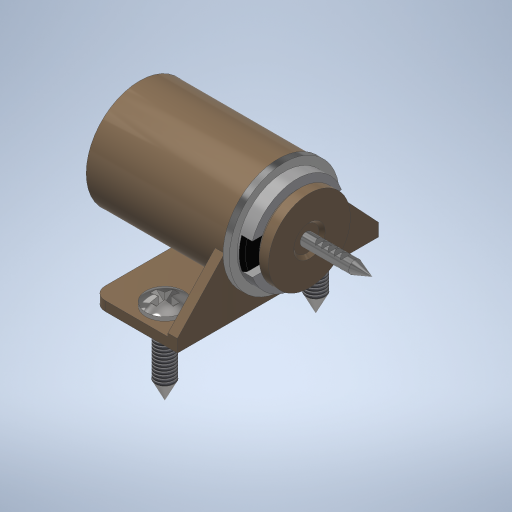
# Autodesk Inventor part: Door fixing magnet
Saved by Autodesk Inventor 2024 (Build 280153000, 153)
## iProperties
Category: Magnets and locks
Created: 2013-04-05
Part Number: Door fixing magnet
Material: Generic
Document SubType Name: Modeling
Designer: G. K.
Authority: Design by UAB Čeli APS
Density: 1 g/cm^3
Description: Door  fixing magnet
Appearance: Default
Mase: 0.0
Author: G. K.
Title: Door fixing magnet
Subject: Magnets
Keywords: door, magnets
Comments: magnet for doors fixing
Revision Number: 1
Autodesk Inventor part; units mm, degrees
sketch "Sketch2" plane through (0, 0, 0) normal (0, 1, 0) x (-1, 0, 0)
  line L0 (0, 0) -> (-25, 0)
  line L1 (0, -7.5) -> (-8, -7.5)
  line L2 (-22, -8.5) -> (0, -8.5)
  line L3 (0, -8.5) -> (0, -7.5)
  line L4 (-8, -7.5) -> (-8, -4)
  line L5 (-8, -4) -> (-2, -4)
  line L6 (-2, -4) -> (-2, 0)
  line L7 (-22, -8.5) -> (-22, -8.75)
  line L8 (-22, -8.75) -> (-23, -8.75)
  line L9 (-23, -8.75) -> (-23, -7.5)
  line L10 (-23, -7.5) -> (-25, -7.5)
  line L11 (-25, -7.5) -> (-25, 0)
  dimension "d0" = 15
  dimension "d2" = 17
  dimension "d3" = 8
  dimension "d4" = 0
  dimension "d5" = 8
  dimension "d6" = 22
  dimension "d7" = 1
  dimension "d8" = 2
  dimension "d9" = 17.5
  dimension "d10" = 15
  dimension "d12" = 23
  constraints: 25 end point, 5 parallel, 5 perpendicular, 1 horizontal, 1 point on line
  measures "d0" diameter of L1 L0
  measures "d2" diameter of L2 L0
  measures "d3" distance between parallel lines of L4 L3
  measures "d4" distance from line of L0.start L3
  measures "d5" diameter of L5 L0
  measures "d6" distance between parallel lines of L7 L3
  measures "d7" distance of L7.end L8.end
  measures "d8" distance of L9.end L10.end
  measures "d9" diameter of L8 L0
  measures "d10" diameter of L10 L0
  measures "d12" distance between parallel lines of L6 L11
revolve "Revolution1" add sketch "Sketch2" angle 360 about axis through (0, 0, 0) along (1, 0, 0)
sketch "Sketch3" plane through (22, 0, 0) normal (-1, 0, 0) x (0, 0, 1)
  circle A0 centre (0, 0) radius 8.75 projected
  line L0 (-10, -16) -> (-10, 16)
  line L1 (-10, 16) -> (-8, 16)
  line L2 (-10, -16) -> (-8, -16)
  circle A1 centre (0, 0) radius 8.5 projected
  line L3 (0, -8.5) -> (-8, -16)
  line L4 (0, 8.5) -> (-8, 16)
  dimension "d14" = 2
  dimension "d16" = 2
  dimension "d18" = 32
  dimension "d19" = 16
  dimension "d22" = 10
  constraints: 10 end point, 2 point on circle, 1 parallel, 1 perpendicular, 1 vertical
  measures "d14" distance of L0.start L2.end
  measures "d16" distance of L0.end L1.end
  measures "d18" distance of L0.start L0.end
  measures "d19" distance from line of A0.centre L2
  measures "d22" distance from line of A0.centre L0
ref_plane "Work Plane3" through (20.5, 0, 0) normal (-1, 0, 0) x (0, 0, 1)
sketch "Sketch4" plane through (20.5, 0, 0) normal (-1, 0, 0) x (0, 0, 1)
  line L0 (-8.5, 16) -> (-8.5, -16)
  line L1 (-8.5, -16) -> (-10, -16)
  line L2 (-10, -16) -> (-10, 16)
  line L3 (-8.5, 16) -> (-10, 16)
  constraints: 8 end point, 2 parallel
extrude "Extrusion2" add sketch "Sketch4" along normal blind 12
sketch "Sketch5" plane through (0, 0, 0) normal (0, 1, 0) x (-1, 0, 0)
  line L0 (-25, 2.4451) -> (-23.8, 2.4451)
  line L1 (-23.8, 2.4451) -> (-23.8, -2.5549)
  line L2 (-23.8, -2.5549) -> (-25, -2.5549)
  line L3 (-25, -2.5549) -> (-25, 2.4451)
  line L4 (-2, 4) -> (-2, -4) projected
  line L5 (-2, -4) -> (-8, -4) projected
  line L6 (-8, -4) -> (-8, -7.5) projected
  line L7 (-8, -7.5) -> (0, -7.5) projected
  line L8 (0, -7.5) -> (0, -8.5) projected
  line L9 (0, -8.5) -> (-8.5, -8.5) projected
  line L10 (-22, -8.75) -> (-23, -8.75) projected
  line L11 (-23, -8.75) -> (-23, -7.5) projected
  line L12 (-23, -7.5) -> (-25, -7.5) projected
  line L13 (-25, -7.5) -> (-25, 7.5) projected
  line L14 (-25, 7.5) -> (-23, 7.5) projected
  line L15 (-23, 7.5) -> (-23, 8.75) projected
  line L16 (-23, 8.75) -> (-22, 8.75) projected
  line L17 (-22, 8.5) -> (0, 8.5) projected
  line L18 (0, 8.5) -> (0, 7.5) projected
  line L19 (0, 7.5) -> (-8, 7.5) projected
  line L20 (-8, 7.5) -> (-8, 4) projected
  line L21 (-8, 4) -> (-2, 4) projected
  line L22 (-2, 4) -> (-2, -4) projected
  line L23 (-2, -4) -> (-8, -4) projected
  line L24 (-8, -4) -> (-8, -7.5) projected
  line L25 (-8, -7.5) -> (0, -7.5) projected
  line L26 (0, -7.5) -> (0, -8.5) projected
  line L27 (0, -8.5) -> (-8.5, -8.5) projected
  line L28 (-22, -8.75) -> (-23, -8.75) projected
  line L29 (-23, -8.75) -> (-23, -7.5) projected
  line L30 (-23, -7.5) -> (-25, -7.5) projected
  line L31 (-25, -7.5) -> (-25, 7.5) projected
  line L32 (-25, 7.5) -> (-23, 7.5) projected
  line L33 (-23, 7.5) -> (-23, 8.75) projected
  line L34 (-23, 8.75) -> (-22, 8.75) projected
  line L35 (-22, 8.5) -> (0, 8.5) projected
  line L36 (0, 8.5) -> (0, 7.5) projected
  line L37 (0, 7.5) -> (-8, 7.5) projected
  line L38 (-8, 7.5) -> (-8, 4) projected
  line L39 (-8, 4) -> (-2, 4) projected
  line L40 (-22, -8.5) -> (-22, -8.75) projected
  line L41 (-22, 8.75) -> (-22, 8.5) projected
  line L42 (-22, -8.5) -> (-22, -8.75) projected
  line L43 (-22, 8.75) -> (-22, 8.5) projected
  line L44 (-8.5, -8.5) -> (-8.5, -10) projected
  line L45 (-20.5, -10) -> (-20.5, -8.5) projected
  line L46 (-20.5, -8.5) -> (-22, -8.5) projected
  line L47 (-20.5, -8.5) -> (-8.5, -8.5) projected
  line L48 (-8.5, -8.5) -> (-8.5, -10) projected
  line L49 (-20.5, -10) -> (-20.5, -8.5) projected
  line L50 (-20.5, -8.5) -> (-22, -8.5) projected
  line L51 (-20.5, -8.5) -> (-8.5, -8.5) projected
  line L52 (-8.5, -10) -> (-20.5, -10) projected
  line L53 (-8.5, -10) -> (-20.5, -10) projected
  point P0 (0, 0)
  point P1 (-25, -0.0549)
  point P2 (-25, 0)
  dimension "d28" = 5
  dimension "d30" = 1.2
  constraints: 8 end point, 2 midpoint, 2 parallel, 1 horizontal, 1 perpendicular, 1 vertical alignment
  measures "d28" distance between parallel lines of L2 L0
  measures "d30" distance of L0.start L0.end
extrude "Extrusion4" cut sketch "Sketch5" along normal through all both and the other way through all contours L0 L1 L2 L3
fillet "Fillet2" radius 0.5 2 edges at (23.8, -7.4998, -0.0583) (23.8, 7.4998, -0.0583)
ref_plane "Work Plane4" through (22, -16, -10) normal (0, 0, -1) x (-1, 0, 0)
sketch "Sketch6" plane through (22, -16, -10) normal (0, 0, -1) x (-1, 0, 0)
  point P0 (22, 16)
  point P1 (6, 4)
  point P2 (6, 28)
  dimension "d38" = 24
  measures "d38" distance of point (6, 28) point (6, 4)
hole "Hole1" at (16, -12, -10) at (16, 12, -10) direction (0, 0, 1) diameter 3.2 end through all
chamfer "Chamfer1" distance 1 angle 45 1 edges at (2, 0, 4)
thread "Thread1" size "M8x1.25" class "6g" standard "ANSI Metric M Profile" full length
sketch "Sketch7" plane through (0, 0, 0) normal (0, 1, 0) x (-1, 0, 0)
  line L0 (0, -7.5) -> (0, -8.5) projected
  line L1 (0, -8.5) -> (-8.5, -8.5) projected
  line L2 (-22, -8.75) -> (-23, -8.75) projected
  line L3 (-23, -8.75) -> (-23, -7.5) projected
  line L4 (-23, -7.5) -> (-25, -7.5) projected
  line L5 (-25, -7.5) -> (-25, -2.5549) projected
  line L6 (-25, -2.5549) -> (-23.8, -2.5549) projected
  line L7 (-23.8, -2.5549) -> (-23.8, 2.4451) projected
  line L8 (-23.8, 2.4451) -> (-25, 2.4451) projected
  line L9 (-25, 2.4451) -> (-25, 7.5) projected
  line L10 (-25, 7.5) -> (-23, 7.5) projected
  line L11 (-23, 7.5) -> (-23, 8.75) projected
  line L12 (-23, 8.75) -> (-22, 8.75) projected
  line L13 (-22, 8.5) -> (0, 8.5) projected
  line L14 (0, 8.5) -> (0, 7.5) projected
  line L15 (0, 7.5) -> (-8, 7.5) projected
  line L16 (-8, 7.5) -> (-8, 4) projected
  line L17 (-8, 4) -> (-3, 4) projected
  line L18 (-3, 4) -> (-2, 3) projected
  line L19 (-2, 3) -> (-2, -3) projected
  line L20 (-2, -3) -> (-3, -4) projected
  line L21 (-3, -4) -> (-8, -4) projected
  line L22 (-8, -4) -> (-8, -7.5) projected
  line L23 (-8, -7.5) -> (0, -7.5) projected
  line L24 (0, 0) -> (-37, 0)
  line L25 (-25, 0) -> (-25, 6.5)
  line L26 (-25, 6.5) -> (-27, 6.5)
  line L27 (-27, 6.5) -> (-27, 2.5)
  line L28 (-27, 2.5) -> (-26.5, 2)
  line L29 (-26.5, 2) -> (-26.5, 1)
  line L30 (-26.5, 1) -> (-34.2525, 1)
  line L31 (-34.2525, 1) -> (-37, 0)
  line L32 (-34.2525, 1) -> (-31.3287, 1) construction
  line L33 (-22, -8.5) -> (-22, -8.75) projected
  line L34 (-22, 8.75) -> (-22, 8.5) projected
  line L35 (-8.5, -8.5) -> (-8.5, -10) projected
  line L36 (-20.5, -10) -> (-20.5, -8.5) projected
  line L37 (-20.5, -8.5) -> (-22, -8.5) projected
  line L38 (-20.5, -8.5) -> (-8.5, -8.5) projected
  line L39 (-8.5, -10) -> (-20.5, -10) projected
  dimension "d52" = 13
  dimension "d54" = 2
  dimension "d55" = 5
  dimension "d56" = 0.5
  dimension "d57" = 4
  dimension "d58" = 2
  dimension "d59" = 160
  dimension "d60" = 12
  constraints: 19 end point, 3 perpendicular, 2 parallel, 2 point on line, 1 equal length, 1 horizontal
  measures "d52" diameter of L26 L24
  measures "d54" distance between parallel lines of L9 L27
  measures "d55" diameter of L27.end L24
  measures "d56" distance from line of L27 L28.end
  measures "d57" diameter of L28.end L24
  measures "d58" diameter of L30 L24
  measures "d59" angle of L31 L32
  measures "d60" distance from line of L24.end L25
revolve "Revolution2" add sketch "Sketch7" angle 360 about axis through (0, 0, 0) along (1, 0, 0) separate body contours L24 L31 L30 L29 L28 L27 L26 L9 L25
ref_plane "Work Plane1" through (0, 10, 0) normal (0, 1, 0) x (-1, 0, 0)
sketch "Sketch10" plane through (0, 10, 0) normal (0, 1, 0) x (-1, 0, 0)
  line L0 (-34.2525, 1) -> (-26.5, 1) construction
  line L1 (-34.2525, -1) -> (-34.2525, 1) construction
  line L2 (-33.1525, 1) -> (-32.7525, 0.6)
  line L3 (-32.7525, 0.6) -> (-32.3525, 1)
  line L4 (-32.7525, 0.6) -> (-32.7525, 1) construction
  line L5 (-33.1525, 1) -> (-32.3525, 1)
  line L6 (-34.2525, 0) -> (-32.9237, 0) construction
  point P0 (0, 0)
  dimension "d73" = 45
  dimension "d74" = 45
  dimension "d75" = 1.5
  dimension "d76" = 0.6
  constraints: 10 end point, 3 point on line, 1 collinear, 1 midpoint, 1 parallel, 1 perpendicular
  measures "d73" angle of L4 L2
  measures "d74" angle of L4 L3
  measures "d75" distance from line of L2.end L1
  measures "d76" distance from line of L2.end L6
extrude "Extrusion5" cut sketch "Sketch10" against normal blind 12 bodies 2
pattern_circular "Circular Pattern1" count 2 over 360 about axis through (30.3763, 0, 0) along (-1, 0, 0) of "Extrusion5" bodies 2
pattern_linear "Rectangular Pattern1" count 5 spacing 1 along (-1, 0, 0) of "Extrusion5", "Circular Pattern1" bodies 2
chamfer "Chamfer2" distance 0.5 angle 45 1 edges at (25, 0, -6.5)
ref_plane "Work Plane2" through (16, -12, 34.7276) normal (-1, 0, 0) x (0, 0, -1)
sketch "Sketch11" plane through (16, -12, 34.7276) normal (-1, 0, 0) x (0, 0, -1)
  line L0 (30.4276, 0) -> (60.5276, 0) projected
  line L1 (42.6276, 3) -> (43.2276, 3)
  line L2 (43.2276, 3) -> (43.2276, 1.5)
  line L3 (43.2276, 1.5) -> (53.2276, 1.5)
  line L4 (53.2276, 1.5) -> (56.2276, 0)
  arc A0 (42.6276, 3) -> (41.8238, 0) centre (47.8238, 0) ccw
  line L5 (48.442, 0) -> (56.2276, 0)
  point P0 (34.7276, -12)
  dimension "d89" = 3
  dimension "d91" = 6
  dimension "d92" = 6
  dimension "d93" = 13
  dimension "d95" = 3
  constraints: 10 end point, 4 point on line, 2 parallel, 2 point on circle, 1 centre point, 1 collinear, 1 perpendicular
  measures "d89" diameter of L3 L0
  measures "d91" diameter of L1 L0
  measures "d92" radius of A0
  measures "d93" distance from line of L4.end L2
  measures "d95" horizontal distance of L3.end L4.end
revolve "Revolution3" add sketch "Sketch11" angle 360 about axis through (16, -12, 34.7276) along (0, 0, -1) separate body
sketch "Sketch13" plane through (16, -12, 34.7276) normal (-1, 0, 0) x (0, 0, -1)
  line L0 (41.7776, 2.222) -> (41.7776, 0)
  line L1 (41.7776, 0) -> (43.2276, 0)
  line L2 (43.2276, 0) -> (43.2276, 0.6)
  line L3 (43.2276, 0.6) -> (41.7776, 2.222)
  point P0 (34.7276, -12)
  dimension "d105" = 0.6
  dimension "d106" = 1.45
  dimension "d107" = 2.222
  constraints: 9 end point, 1 parallel, 1 perpendicular, 1 vertical
  measures "d105" distance of L1.end L2.end
  measures "d106" distance between parallel lines of L2 L0
  measures "d107" distance of L0.start L0.end
extrude "Extrusion8" cut sketch "Sketch13" along normal mid plane 1 bodies 3
pattern_circular "Circular Pattern2" count 4 over 360 about axis through (16, -12, -13.5) along (0, 0, -1) of "Extrusion8" bodies 3
thread "Thread2" size "M3x0.5" class "6g" standard "ANSI Metric M Profile" length 8
extrude "Extrusion9" add sketch "Sketch3" along normal blind 1.5 contours L4 A1 L3 A0 | A0 L3 L2 L0 L1 L4 picked at (-0.7655, -8.4997) bodies 1
pattern_linear "Rectangular Pattern3" count 2 spacing 24 along (0, 1, 0) bodies 3
fillet "Fillet3" radius 2 2 edges at (8.5, -16, -9.25) (8.5, 16, -9.25)
